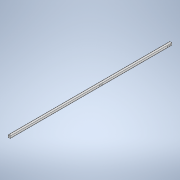
# Autodesk Inventor part: プレート保持_角柱1
Saved by Autodesk Inventor 2021 (Build 250183000, 183)
## iProperties
Created: 2022-02-03
Part Number: プレート保持_角柱1
Material: 一般
Document SubType Name: Modeling
Designer: hirohumi
Density: 1 g/cm^3
Appearance: 既定
Author: hirohumi
Autodesk Inventor part; units mm, degrees
ref_plane "YZ Plane" through (0, 0, 0) normal (1, 0, 0) x (0, 1, 0)
ref_plane "XZ Plane" through (0, 0, 0) normal (0, 1, 0) x (-1, 0, 0)
ref_plane "XY Plane" through (0, 0, 0) normal (0, 0, 1) x (1, 0, 0)
sketch "スケッチ1" plane through (0, 0, 0) normal (0, 0, 1) x (1, 0, 0)
  line L0 (7.5, 7.5) -> (-7.5, 7.5)
  line L1 (-7.5, 7.5) -> (-7.5, -7.5)
  line L2 (-7.5, -7.5) -> (7.5, -7.5)
  line L3 (7.5, -7.5) -> (7.5, 7.5)
  line L4 (7.5, 7.5) -> (-7.5, -7.5) construction
  line L5 (-7.5, 7.5) -> (7.5, -7.5) construction
  line L6 (-6.5, 6.5) -> (6.5, 6.5)
  line L7 (6.5, 6.5) -> (6.5, -6.5)
  line L8 (6.5, -6.5) -> (-6.5, -6.5)
  line L9 (-6.5, -6.5) -> (-6.5, 6.5)
  point P0 (0, 0)
  dimension "d0" = 15
  dimension "d1" = 15
  dimension "d2" = 1
  constraints: 20 end point, 4 parallel, 2 midpoint, 2 perpendicular, 1 horizontal, 3 other
  measures "d0" distance of L2.end L1.end
  measures "d1" distance of L1.end L0.end
  measures "d2" distance between parallel lines of L0 L6
extrude "押し出し1" add sketch "スケッチ1" along normal blind 1142
sketch "スケッチ2" plane through (7.5, 7.5, 1142) normal (1, 0, 0) x (0, 0, -1)
  circle A0 centre (1132, -7.5) radius 1.6
  circle A1 centre (1122, -7.5) radius 1.6
  circle A2 centre (1112, -7.5) radius 1.6
  line L0 (1142, -15) -> (1142, 0) projected
  circle A3 centre (652, -7.5) radius 1.6
  circle A4 centre (642, -7.5) radius 1.6
  circle A5 centre (632, -7.5) radius 1.6
  point P0 (1142, -7.5)
  point P1 (1142, -7.5)
  dimension "d5" = 3.2
  dimension "d6" = 3.2
  dimension "d7" = 3.2
  dimension "d8" = 10
  dimension "d9" = 10
  dimension "d10" = 10
  dimension "d11" = 3.2
  dimension "d12" = 3.2
  dimension "d13" = 3.2
  dimension "d14" = 10
  dimension "d15" = 10
  dimension "d16" = 500
  constraints: 6 centre point, 6 horizontal alignment, 1 midpoint
  measures "d5" diameter of A0
  measures "d6" diameter of A1
  measures "d7" diameter of A2
  measures "d8" distance of point (1142, -7.5) A0.centre
  measures "d9" distance of A0.centre A1.centre
  measures "d10" distance of A1.centre A2.centre
  measures "d11" diameter of A3
  measures "d12" diameter of A4
  measures "d13" diameter of A5
  measures "d14" distance of A3.centre A4.centre
  measures "d15" distance of A4.centre A5.centre
  measures "d16" distance of point (1142, -7.5) A4.centre
extrude "押し出し2" cut sketch "スケッチ2" against normal through all
sketch "スケッチ3" plane through (-7.5, 7.5, 1142) normal (0, 1, 0) x (1, 0, 0)
  circle A0 centre (7.5, 7.5) radius 1.6
  line L0 (0, 1142) -> (0, 0) projected
  line L1 (15, 0) -> (0, 0) projected
  point P0 (7.5, 1142)
  dimension "d19" = 3.2
  dimension "d20" = 7.5
  dimension "d21" = 7.5
  constraints: 1 centre point
  measures "d19" diameter of A0
  measures "d20" distance from line of L0 A0.centre
  measures "d21" distance from line of L1 A0.centre
extrude "押し出し3" cut sketch "スケッチ3" against normal through all
